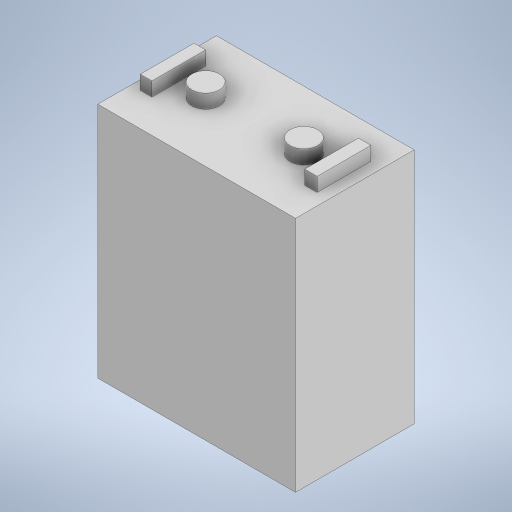
# Autodesk Inventor part: battery
Saved by Autodesk Inventor 2023 (Build 270158000, 158)
## iProperties
Created: 2022-06-19
Part Number: battery
Material: Generic
Document SubType Name: Modeling
Designer: ADITYA CHINAGUDI
Density: 1 g/cm^3
Appearance: Default
Author: ADITYA CHINAGUDI
Autodesk Inventor part; units mm, degrees
ref_plane "YZ Plane" through (0, 0, 0) normal (1, 0, 0) x (0, 1, 0)
ref_plane "XZ Plane" through (0, 0, 0) normal (0, 1, 0) x (-1, 0, 0)
ref_plane "XY Plane" through (0, 0, 0) normal (0, 0, 1) x (1, 0, 0)
sketch "Sketch1" plane through (0, 0, 0) normal (0, 0, 1) x (1, 0, 0)
  point P0 (0, 0)
sketch "Sketch2" plane through (0, 0, 0) normal (0, 0, 1) x (1, 0, 0)
  line L0 (-9.8946, 8.2346) -> (40.1054, 8.2346)
  line L1 (40.1054, 8.2346) -> (40.1054, -51.7654)
  line L2 (40.1054, -51.7654) -> (-9.8946, -51.7654)
  line L3 (-9.8946, -51.7654) -> (-9.8946, 8.2346)
  point P0 (0, 0)
  dimension "d0" = 50
  dimension "d1" = 60
  constraints: 8 end point, 2 parallel, 1 horizontal, 1 perpendicular
  measures "d0" distance of L1.end L2.end
  measures "d1" distance of L0.end L1.end
extrude "Extrusion1" add sketch "Sketch2" along normal blind 30
sketch "Sketch3" plane through (-9.8946, 8.2346, 0) normal (0, 1, 0) x (1, 0, 0)
  line L0 (2.3069, -21.5805) -> (5.2632, -21.5805)
  line L1 (5.2632, -21.5805) -> (5.2632, -7.9818)
  line L2 (5.2632, -7.9818) -> (2.3069, -7.9818)
  line L3 (2.3069, -7.9818) -> (2.3069, -21.5805)
  line L4 (43.8913, -21.5805) -> (47.0446, -21.5805)
  line L5 (47.0446, -21.5805) -> (47.0446, -7.9818)
  line L6 (47.0446, -7.9818) -> (43.8913, -7.9818)
  line L7 (43.8913, -7.9818) -> (43.8913, -21.5805)
  point P0 (9.8946, 0)
  constraints: 16 end point, 4 parallel, 2 horizontal, 2 perpendicular, 2 point on line
extrude "Extrusion2" add sketch "Sketch3" along normal blind 3.5
sketch "Sketch4" plane through (-9.8946, 8.2346, 0) normal (0, 1, 0) x (1, 0, 0)
  circle A0 centre (12.2632, -15) radius 3.5
  line L0 (50, -30) -> (0, -30) projected
  circle A1 centre (36.8913, -14.7812) radius 3.5
  line L1 (5.2632, -21.5805) -> (5.2632, -7.9818) projected
  line L2 (43.8913, -7.9818) -> (43.8913, -21.5805) projected
  point P0 (9.8946, 0)
  point P1 (5.2632, -14.7812)
  point P2 (43.8913, -14.7812)
  dimension "d6" = 15
  dimension "d7" = 7
  dimension "d8" = 7
  dimension "d9" = 7
  dimension "d10" = 24.6281
  dimension "d11" = 7
  constraints: 2 centre point, 2 midpoint
  measures "d6" distance from line of A0.centre L0
  measures "d7" horizontal distance of A0.centre point (5.263, -14.781)
  measures "d8" distance of point (43.891, -14.781) A1.centre
  measures "d9" diameter of A1
  measures "d10" horizontal distance of A1.centre A0.centre
  measures "d11" diameter of A0
extrude "Extrusion3" add sketch "Sketch4" along normal blind 3.5
body "Solid1"
